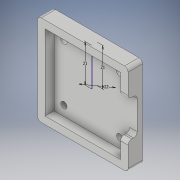
# Autodesk Inventor part: Yaw Shaft Mount
Saved by Autodesk Inventor 2019 (Build 230136000, 136)
## iProperties
Created: 2018-05-28
Part Number: Yaw Shaft Mount
Material: Generic
Document SubType Name: Modeling
Designer: samps
Density: 1 g/cm^3
Appearance: Default
Author: samps
Autodesk Inventor part; units mm, degrees
ref_plane "YZ Plane" through (0, 0, 0) normal (1, 0, 0) x (0, 1, 0)
ref_plane "XZ Plane" through (0, 0, 0) normal (0, 1, 0) x (-1, 0, 0)
ref_plane "XY Plane" through (0, 0, 0) normal (0, 0, 1) x (1, 0, 0)
sketch "Sketch1" plane through (0, 0, 0) normal (0, 0, 1) x (1, 0, 0)
  line L0 (0, 0) -> (42, 0)
  line L1 (42, 0) -> (42, -42)
  line L2 (42, -42) -> (0, -42)
  line L3 (0, -42) -> (0, 0)
  line L4 (0, 0) -> (-1, 0)
  line L5 (-1, 0) -> (-4.175, 0)
  line L6 (-4.175, 0) -> (-4.175, 1)
  line L7 (-4.175, 1) -> (-4.175, 4.175)
  line L8 (-4.175, 4.175) -> (42, 4.175)
  line L9 (42, 4.175) -> (43, 4.175)
  line L10 (43, 4.175) -> (46.175, 4.175)
  line L11 (-4.175, 4.175) -> (46.175, 4.175)
  line L12 (46.175, 4.175) -> (46.175, -46.175)
  line L13 (46.175, -46.175) -> (-4.175, -46.175)
  line L14 (-4.175, -46.175) -> (-4.175, 4.175)
  dimension "d0" = 42
  dimension "d1" = 42
  dimension "d2" = 1
  dimension "d3" = 3.175
  dimension "d4" = 1
  dimension "d5" = 3.175
  dimension "d6" = 1
  dimension "d7" = 3.175
  dimension "d8" = 50.35
  constraints: 30 end point, 4 parallel, 4 perpendicular, 3 horizontal, 3 point on line, 1 vertical
  measures "d0" distance of L1.end L2.end
  measures "d1" distance of L0.end L1.end
  measures "d2" distance of L0.start L4.end
  measures "d3" distance of L4.end L5.end
  measures "d4" distance of L5.end L6.end
  measures "d5" distance of L6.end L7.end
  measures "d6" distance of L8.end L9.end
  measures "d7" distance of L9.end L10.end
  measures "d8" distance of L11.end L12.end
extrude "Extrusion1" add sketch "Sketch1" along normal blind 8
sketch "Sketch2" plane through (0, 0, 0) normal (0, 0, -1) x (-1, 0, 0)
  line L0 (0, -42) -> (0, 0) projected
  line L1 (-42, 0) -> (-42, -42) projected
  line L2 (0, 0) -> (-42, 0)
  line L3 (-42, 0) -> (-42, -42)
  line L4 (-42, -42) -> (0, -42)
  line L5 (0, -42) -> (0, 0)
  constraints: 8 end point, 2 parallel, 1 horizontal, 1 perpendicular
extrude "Extrusion2" add sketch "Sketch2" against normal blind 3
sketch "Sketch3" plane through (0, 0, 3) normal (0, 0, 1) x (1, 0, 0)
  line L0 (0, -42) -> (0, 0) projected
  line L1 (0, -42) -> (21, -42)
  line L2 (42, 0) -> (42, -42) projected
  line L3 (21, -42) -> (21, -21)
  line L4 (21, -21) -> (21, -36.5)
  line L5 (21, -36.5) -> (36.5, -36.5)
  line L6 (36.5, -36.5) -> (5.5, -36.5)
  line L7 (5.5, -36.5) -> (5.5, -5.5)
  line L8 (5.5, -5.5) -> (36.5, -5.5)
  line L9 (36.5, -5.5) -> (36.5, -36.5)
  dimension "d13" = 21
  dimension "d14" = 21
  dimension "d15" = 15.5
  dimension "d16" = 15.5
  dimension "d17" = 31
  dimension "d18" = 31
  constraints: 16 end point, 4 perpendicular, 2 parallel, 1 horizontal, 1 point on line
  measures "d13" distance of L0.start L1.end
  measures "d14" distance of L1.end L3.end
  measures "d15" distance of L3.end L4.end
  measures "d16" distance of L4.end L5.end
  measures "d17" distance of L7.end L8.end
  measures "d18" distance of L6.end L7.end
hole "Hole1" at (5.5, -5.5, 3) at (36.5, -5.5, 3) at (36.5, -36.5, 3) at (5.5, -36.5, 3) direction (0, 0, -1) diameter 3.5 depth 3.5
sketch "Sketch4" plane through (46.175, -46.175, 0) normal (1, 0, 0) x (0, 0, -1)
  line L0 (0, 0) -> (0, 50.35) projected
  line L1 (0, 25.175) -> (-3, 25.175)
  line L2 (-3, 46.175) -> (-3, 4.175) projected
  line L3 (-3, 25.175) -> (-3, 15.175)
  line L4 (-8, 46.175) -> (-8, 4.175) projected
  line L5 (-3, 15.175) -> (-8, 15.175)
  line L6 (-8, 15.175) -> (-8, 35.175)
  line L7 (-8, 35.175) -> (-3, 35.175)
  line L8 (-3, 35.175) -> (-3, 15.175)
  point P0 (0, 46.175)
  dimension "d26" = 10
  dimension "d27" = 20
  constraints: 12 end point, 2 midpoint, 2 parallel, 2 point on line, 1 horizontal, 1 perpendicular
  measures "d26" distance of L1.end L3.end
  measures "d27" distance of L5.end L6.end
extrude "Extrusion3" cut sketch "Sketch4" against normal blind 5
fillet "Fillet1" radius 2 8 edges at (44.0875, -11, 3) (44.0875, -31, 3) (44.0875, -11, 8) (44.0875, -31, 8) (46.175, 4.175, 4) (46.175, -46.175, 4) (-4.175, -46.175, 4) (-4.175, 4.175, 4)
sketch "Sketch5" plane through (0, 0, 3) normal (0, 0, 1) x (1, 0, 0)
  line L0 (42, 0) -> (42, -9) projected
  line L1 (42, 0) -> (21, 0)
  line L2 (0, 0) -> (42, 0) projected
  line L3 (21, 0) -> (21, -21)
  dimension "d31" = 21
  constraints: 4 end point, 1 midpoint, 1 vertical
  measures "d31" distance of L1.end L3.end
sketch "Sketch6" plane through (0, 0, 0) normal (0, 0, -1) x (-1, 0, 0)
  line L0 (0, 0) -> (-42, 0) projected
  line L1 (-21, 0) -> (-21, -21)
  circle A0 centre (-21, -21) radius 11
  dimension "d32" = 21
  dimension "d33" = 22
  constraints: 2 end point, 1 centre point, 1 coincident, 1 midpoint, 1 vertical
  measures "d32" distance of L1.start L1.end
  measures "d33" diameter of A0
body "Solid1"
